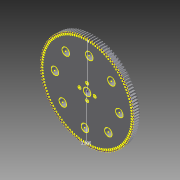
# Autodesk Inventor part: 120 tooth gear
Saved by Autodesk Inventor 2015 (Build 190159000, 159)
## iProperties
Created: 2011-10-31
Part Number: 120 tooth gear
Material: Generic
Document SubType Name: Modeling
Designer: Kyle
Density: 1 g/cm^3
Appearance: Default
Author: Kyle
Autodesk Inventor part; units mm, degrees
ref_plane "YZ Plane" through (0, 0, 0) normal (1, 0, 0) x (0, 1, 0)
ref_plane "XZ Plane" through (0, 0, 0) normal (0, 1, 0) x (-1, 0, 0)
ref_plane "XY Plane" through (0, 0, 0) normal (0, 0, 1) x (1, 0, 0)
sketch "Sketch1" plane through (0, 0, 0) normal (0, 0, 1) x (1, 0, 0)
  circle A0 centre (0, 0) radius 46.0375
  circle A1 centre (0, 0) radius 3.9688
  circle A2 centre (0, 7.9375) radius 1.5875
  circle A3 centre (-7.9375, 0) radius 1.5875
  circle A4 centre (0, -7.9375) radius 1.5875
  circle A5 centre (7.9375, 0) radius 1.5875
  circle A6 centre (25.4, 22.225) radius 3.9688
  circle A7 centre (0, 0) radius 3.9688
  circle A8 centre (2.2451, 33.676) radius 3.9688
  circle A9 centre (0, 0) radius 3.9688
  circle A10 centre (-22.225, 25.4) radius 3.9688
  circle A11 centre (0, 0) radius 3.9688
  circle A12 centre (-33.676, 2.2451) radius 3.9688
  circle A13 centre (0, 0) radius 3.9688
  circle A14 centre (-25.4, -22.225) radius 3.9688
  circle A15 centre (0, 0) radius 3.9688
  circle A16 centre (-2.2451, -33.676) radius 3.9688
  circle A17 centre (0, 0) radius 3.9688
  circle A18 centre (22.225, -25.4) radius 3.9688
  circle A19 centre (0, 0) radius 3.9688
  circle A20 centre (33.676, -2.2451) radius 3.9688
  dimension "d0" = 92.075
  dimension "d1" = 7.9375
  dimension "d2" = 3.175
  dimension "d3" = 7.9375
  dimension "d6" = 360
  dimension "d8" = 7.9375
  dimension "d9" = 22.225
  dimension "d10" = 25.4
  dimension "d13" = 360
  constraints: 21 centre point, 4 coincident, 40 other
  measures "d0" diameter of A0
  measures "d1" diameter of A1
  measures "d2" diameter of A2
  measures "d3" distance of A1.centre A2.centre
  measures "d8" diameter of A6
  measures "d9" vertical distance of A1.centre A6.centre
  measures "d10" horizontal distance of A1.centre A6.centre
extrude "Extrusion1" add sketch "Sketch1" along normal blind 6.35
sketch "Sketch2" plane through (0, 0, 6.35) normal (0, 0, 1) x (1, 0, 0)
  circle A0 centre (0, 0) radius 46.0375 projected
  line L0 (0, 46.0375) -> (0, 48.6765) construction
  line L1 (0, 48.6765) -> (0.3969, 48.6765)
  line L2 (0.3969, 48.6765) -> (0.7937, 47.089)
  line L3 (0.7937, 47.089) -> (0.7938, 46.0307)
  line L4 (0, 48.6765) -> (-0.3969, 48.6765)
  line L5 (-0.3969, 48.6765) -> (-0.7938, 47.089)
  line L6 (-0.7938, 47.089) -> (-0.7938, 46.0307)
  arc A1 (0.7938, 46.0307) -> (-0.7938, 46.0307) centre (0, 0) ccw
  dimension "d17" = 0.3969
  dimension "d18" = 1.5875
  dimension "d19" = 0.3969
  dimension "d20" = 1.0583
  constraints: 14 end point, 4 point on circle, 3 symmetric about line, 2 perpendicular, 1 centre point, 1 coincident, 1 concentric, 1 vertical
  measures "d17" distance of L0.end L1.end
  measures "d18" vertical distance of L1.end L2.end
  measures "d19" horizontal distance of L1.end L2.end
  measures "d20" distance of L2.end L3.end
extrude "Extrusion2" add sketch "Sketch2" against normal blind 6.35 contours A0 L6 L5 L4 L1 L2 L3
pattern_circular "Circular Pattern1" count 120 over 360 about axis through (0, 0, 0) along (0, 0, 1) of "Extrusion2"
sketch "Sketch3" plane through (0, 0, 6.35) normal (0, 0, 1) x (1, 0, 0)
  circle A0 centre (33.676, -2.2451) radius 3.9687 projected
  circle A1 centre (22.225, -25.4) radius 3.9687 projected
  circle A2 centre (-2.2451, -33.676) radius 3.9687 projected
  circle A3 centre (-25.4, -22.225) radius 3.9687 projected
  circle A4 centre (-33.676, 2.2451) radius 3.9687 projected
  circle A5 centre (-22.225, 25.4) radius 3.9687 projected
  circle A6 centre (2.2451, 33.676) radius 3.9687 projected
  circle A7 centre (25.4, 22.225) radius 3.9687 projected
  circle A8 centre (0, 0) radius 3.9687 projected
  circle A9 centre (7.9375, 0) radius 1.5875 projected
  circle A10 centre (0, -7.9375) radius 1.5875 projected
  circle A11 centre (-7.9375, 0) radius 1.5875 projected
  circle A12 centre (0, 7.9375) radius 1.5875 projected
  arc A13 (1.6164, 46.0091) -> (0.7938, 46.0307) centre (0, 0) ccw projected
  line L0 (0.7937, 47.089) -> (0.7938, 46.0307) projected
  line L1 (0.3969, 48.6765) -> (0.7937, 47.089) projected
  line L2 (-0.3969, 48.6765) -> (0.3969, 48.6765) projected
  line L3 (-0.7938, 47.089) -> (-0.3969, 48.6765) projected
  line L4 (-0.7938, 46.0307) -> (-0.7938, 47.089) projected
  arc A14 (-0.7938, 46.0307) -> (-1.6164, 46.0091) centre (0, 0) ccw projected
  line L5 (-1.6718, 47.066) -> (-1.6164, 46.0091) projected
  line L6 (-2.1512, 48.6306) -> (-1.6718, 47.066) projected
  line L7 (-2.9439, 48.589) -> (-2.1512, 48.6306) projected
  line L8 (-3.2571, 46.9829) -> (-2.9439, 48.589) projected
  line L9 (-3.2017, 45.926) -> (-3.2571, 46.9829) projected
  arc A15 (-3.2017, 45.926) -> (-4.0221, 45.8615) centre (0, 0) ccw projected
  line L10 (-4.1327, 46.914) -> (-4.0221, 45.8615) projected
  line L11 (-4.6934, 48.4513) -> (-4.1327, 46.914) projected
  line L12 (-5.4828, 48.3684) -> (-4.6934, 48.4513) projected
  line L13 (-5.7115, 46.7481) -> (-5.4828, 48.3684) projected
  line L14 (-5.6009, 45.6955) -> (-5.7115, 46.7481) projected
  arc A16 (-5.6009, 45.6955) -> (-6.4168, 45.5881) centre (0, 0) ccw projected
  line L15 (-6.5824, 46.6334) -> (-6.4168, 45.5881) projected
  line L16 (-7.2227, 48.1393) -> (-6.5824, 46.6334) projected
  line L17 (-8.0067, 48.0151) -> (-7.2227, 48.1393) projected
  line L18 (-8.1503, 46.3851) -> (-8.0067, 48.0151) projected
  line L19 (-7.9848, 45.3398) -> (-8.1503, 46.3851) projected
  arc A17 (-7.9848, 45.3398) -> (-8.7939, 45.1898) centre (0, 0) ccw projected
  line L20 (-9.0139, 46.225) -> (-8.7939, 45.1898) projected
  line L21 (-9.7322, 47.6953) -> (-9.0139, 46.225) projected
  line L22 (-10.5086, 47.5303) -> (-9.7322, 47.6953) projected
  line L23 (-10.5668, 45.895) -> (-10.5086, 47.5303) projected
  line L24 (-10.3467, 44.8597) -> (-10.5668, 45.895) projected
  arc A18 (-10.3467, 44.8597) -> (-11.1469, 44.6676) centre (0, 0) ccw projected
  line L25 (-11.4208, 45.6899) -> (-11.1469, 44.6676) projected
  line L26 (-12.2151, 47.1206) -> (-11.4208, 45.6899) projected
  line L27 (-12.9818, 46.9152) -> (-12.2151, 47.1206) projected
  line L28 (-12.9542, 45.279) -> (-12.9818, 46.9152) projected
  line L29 (-12.6803, 44.2568) -> (-12.9542, 45.279) projected
  arc A19 (-12.6803, 44.2568) -> (-13.4694, 44.023) centre (0, 0) ccw projected
  line L30 (-13.7964, 45.0296) -> (-13.4694, 44.023) projected
  line L31 (-14.6644, 46.4167) -> (-13.7964, 45.0296) projected
  line L32 (-15.4193, 46.1715) -> (-14.6644, 46.4167) projected
  line L33 (-15.3062, 44.539) -> (-15.4193, 46.1715) projected
  line L34 (-14.9792, 43.5325) -> (-15.3062, 44.539) projected
  arc A20 (-14.9792, 43.5325) -> (-15.7549, 43.2578) centre (0, 0) ccw projected
  line L35 (-16.1342, 44.2458) -> (-15.7549, 43.2578) projected
  line L36 (-17.0736, 45.5856) -> (-16.1342, 44.2458) projected
  line L37 (-17.8146, 45.3012) -> (-17.0736, 45.5856) projected
  line L38 (-17.6162, 43.6769) -> (-17.8146, 45.3012) projected
  line L39 (-17.2369, 42.6889) -> (-17.6162, 43.6769) projected
  arc A21 (-17.2369, 42.6889) -> (-17.9972, 42.3739) centre (0, 0) ccw projected
  line L40 (-18.4277, 43.3408) -> (-17.9972, 42.3739) projected
  line L41 (-19.4359, 44.6296) -> (-18.4277, 43.3408) projected
  line L42 (-20.1611, 44.3068) -> (-19.4359, 44.6296) projected
  line L43 (-19.8779, 42.6951) -> (-20.1611, 44.3068) projected
  line L44 (-19.4475, 41.7283) -> (-19.8779, 42.6951) projected
  arc A22 (-19.4475, 41.7283) -> (-20.1902, 41.374) centre (0, 0) ccw projected
  line L45 (-20.6707, 42.317) -> (-20.1902, 41.374) projected
  line L46 (-21.745, 43.5512) -> (-20.6707, 42.317) projected
  line L47 (-22.4523, 43.1909) -> (-21.745, 43.5512) projected
  line L48 (-22.0852, 41.5962) -> (-22.4523, 43.1909) projected
  line L49 (-21.6047, 40.6533) -> (-22.0852, 41.5962) projected
  arc A23 (-21.6047, 40.6533) -> (-22.3279, 40.2606) centre (0, 0) ccw projected
  line L50 (-22.8571, 41.1771) -> (-22.3279, 40.2606) projected
  line L51 (-23.9945, 42.3535) -> (-22.8571, 41.1771) projected
  line L52 (-24.6819, 41.9566) -> (-23.9945, 42.3535) projected
  line L53 (-24.2319, 40.3834) -> (-24.6819, 41.9566) projected
  line L54 (-23.7027, 39.4668) -> (-24.2319, 40.3834) projected
  arc A24 (-23.7027, 39.4668) -> (-24.4044, 39.0369) centre (0, 0) ccw projected
  line L55 (-24.9808, 39.9245) -> (-24.4044, 39.0369) projected
  line L56 (-26.1783, 41.0397) -> (-24.9808, 39.9245) projected
  line L57 (-26.844, 40.6074) -> (-26.1783, 41.0397) projected
  line L58 (-26.3122, 39.0598) -> (-26.844, 40.6074) projected
  line L59 (-25.7358, 38.1722) -> (-26.3122, 39.0598) projected
  arc A25 (-25.7358, 38.1722) -> (-26.414, 37.7061) centre (0, 0) ccw projected
  line L60 (-27.0361, 38.5623) -> (-26.414, 37.7061) projected
  line L61 (-28.2902, 39.6134) -> (-27.0361, 38.5623) projected
  line L62 (-28.9324, 39.1468) -> (-28.2902, 39.6134) projected
  line L63 (-28.3204, 37.6292) -> (-28.9324, 39.1468) projected
  line L64 (-27.6983, 36.773) -> (-28.3204, 37.6292) projected
  arc A26 (-27.6983, 36.773) -> (-28.3512, 36.2721) centre (0, 0) ccw projected
  line L65 (-29.0172, 37.0945) -> (-28.3512, 36.2721) projected
  line L66 (-30.3247, 38.0785) -> (-29.0172, 37.0945) projected
  line L67 (-30.9415, 37.579) -> (-30.3247, 38.0785) projected
  line L68 (-30.2509, 36.0955) -> (-30.9415, 37.579) projected
  line L69 (-29.5849, 35.273) -> (-30.2509, 36.0955) projected
  arc A27 (-29.5849, 35.273) -> (-30.2107, 34.7386) centre (0, 0) ccw projected
  line L70 (-30.9188, 35.5251) -> (-30.2107, 34.7386) projected
  line L71 (-32.276, 36.4392) -> (-30.9188, 35.5251) projected
  line L72 (-32.8659, 35.9081) -> (-32.276, 36.4392) projected
  line L73 (-32.0986, 34.4628) -> (-32.8659, 35.9081) projected
  line L74 (-31.3904, 33.6763) -> (-32.0986, 34.4628) projected
  arc A28 (-31.3904, 33.6763) -> (-31.9873, 33.1099) centre (0, 0) ccw projected
  line L75 (-32.7357, 33.8582) -> (-31.9873, 33.1099) projected
  line L76 (-34.1388, 34.7001) -> (-32.7357, 33.8582) projected
  line L77 (-34.7001, 34.1388) -> (-34.1388, 34.7001) projected
  line L78 (-33.8582, 32.7357) -> (-34.7001, 34.1388) projected
  line L79 (-33.1099, 31.9873) -> (-33.8582, 32.7357) projected
  arc A29 (-33.1099, 31.9873) -> (-33.6763, 31.3904) centre (0, 0) ccw projected
  line L80 (-34.4628, 32.0986) -> (-33.6763, 31.3904) projected
  line L81 (-35.9081, 32.8659) -> (-34.4628, 32.0986) projected
  line L82 (-36.4392, 32.276) -> (-35.9081, 32.8659) projected
  line L83 (-35.5251, 30.9188) -> (-36.4392, 32.276) projected
  line L84 (-34.7386, 30.2107) -> (-35.5251, 30.9188) projected
  arc A30 (-34.7386, 30.2107) -> (-35.273, 29.5849) centre (0, 0) ccw projected
  line L85 (-36.0955, 30.2509) -> (-35.273, 29.5849) projected
  line L86 (-37.579, 30.9415) -> (-36.0955, 30.2509) projected
  line L87 (-38.0785, 30.3247) -> (-37.579, 30.9415) projected
  line L88 (-37.0945, 29.0172) -> (-38.0785, 30.3247) projected
  line L89 (-36.2721, 28.3512) -> (-37.0945, 29.0172) projected
  arc A31 (-36.2721, 28.3512) -> (-36.773, 27.6983) centre (0, 0) ccw projected
  line L90 (-37.6292, 28.3204) -> (-36.773, 27.6983) projected
  line L91 (-39.1468, 28.9324) -> (-37.6292, 28.3204) projected
  line L92 (-39.6134, 28.2902) -> (-39.1468, 28.9324) projected
  line L93 (-38.5623, 27.0361) -> (-39.6134, 28.2902) projected
  line L94 (-37.7061, 26.414) -> (-38.5623, 27.0361) projected
  arc A32 (-37.7061, 26.414) -> (-38.1722, 25.7358) centre (0, 0) ccw projected
  line L95 (-39.0598, 26.3122) -> (-38.1722, 25.7358) projected
  line L96 (-40.6074, 26.844) -> (-39.0598, 26.3122) projected
  line L97 (-41.0397, 26.1783) -> (-40.6074, 26.844) projected
  line L98 (-39.9245, 24.9808) -> (-41.0397, 26.1783) projected
  line L99 (-39.0369, 24.4044) -> (-39.9245, 24.9808) projected
  arc A33 (-39.0369, 24.4044) -> (-39.4668, 23.7027) centre (0, 0) ccw projected
  line L100 (-40.3834, 24.2319) -> (-39.4668, 23.7027) projected
  line L101 (-41.9566, 24.6819) -> (-40.3834, 24.2319) projected
  line L102 (-42.3535, 23.9945) -> (-41.9566, 24.6819) projected
  line L103 (-41.1771, 22.8571) -> (-42.3535, 23.9945) projected
  line L104 (-40.2606, 22.3279) -> (-41.1771, 22.8571) projected
  arc A34 (-40.2606, 22.3279) -> (-40.6533, 21.6047) centre (0, 0) ccw projected
  line L105 (-41.5962, 22.0852) -> (-40.6533, 21.6047) projected
  line L106 (-43.1909, 22.4523) -> (-41.5962, 22.0852) projected
  line L107 (-43.5512, 21.745) -> (-43.1909, 22.4523) projected
  line L108 (-42.317, 20.6707) -> (-43.5512, 21.745) projected
  line L109 (-41.374, 20.1902) -> (-42.317, 20.6707) projected
  arc A35 (-41.374, 20.1902) -> (-41.7283, 19.4475) centre (0, 0) ccw projected
  line L110 (-42.6951, 19.8779) -> (-41.7283, 19.4475) projected
  line L111 (-44.3068, 20.1611) -> (-42.6951, 19.8779) projected
  line L112 (-44.6296, 19.4359) -> (-44.3068, 20.1611) projected
  line L113 (-43.3408, 18.4277) -> (-44.6296, 19.4359) projected
  line L114 (-42.3739, 17.9972) -> (-43.3408, 18.4277) projected
  arc A36 (-42.3739, 17.9972) -> (-42.6889, 17.2369) centre (0, 0) ccw projected
  line L115 (-43.6769, 17.6162) -> (-42.6889, 17.2369) projected
  line L116 (-45.3012, 17.8146) -> (-43.6769, 17.6162) projected
  line L117 (-45.5856, 17.0736) -> (-45.3012, 17.8146) projected
  line L118 (-44.2458, 16.1342) -> (-45.5856, 17.0736) projected
  line L119 (-43.2578, 15.7549) -> (-44.2458, 16.1342) projected
  arc A37 (-43.2578, 15.7549) -> (-43.5325, 14.9792) centre (0, 0) ccw projected
  line L120 (-44.539, 15.3062) -> (-43.5325, 14.9792) projected
  line L121 (-46.1715, 15.4193) -> (-44.539, 15.3062) projected
  line L122 (-46.4167, 14.6644) -> (-46.1715, 15.4193) projected
  line L123 (-45.0296, 13.7964) -> (-46.4167, 14.6644) projected
  line L124 (-44.023, 13.4694) -> (-45.0296, 13.7964) projected
  arc A38 (-44.023, 13.4694) -> (-44.2568, 12.6803) centre (0, 0) ccw projected
  line L125 (-45.279, 12.9542) -> (-44.2568, 12.6803) projected
  line L126 (-46.9152, 12.9818) -> (-45.279, 12.9542) projected
  line L127 (-47.1206, 12.2151) -> (-46.9152, 12.9818) projected
  line L128 (-45.6899, 11.4208) -> (-47.1206, 12.2151) projected
  line L129 (-44.6676, 11.1469) -> (-45.6899, 11.4208) projected
  arc A39 (-44.6676, 11.1469) -> (-44.8597, 10.3467) centre (0, 0) ccw projected
  line L130 (-45.895, 10.5668) -> (-44.8597, 10.3467) projected
  line L131 (-47.5303, 10.5086) -> (-45.895, 10.5668) projected
  line L132 (-47.6953, 9.7322) -> (-47.5303, 10.5086) projected
  line L133 (-46.225, 9.0139) -> (-47.6953, 9.7322) projected
  line L134 (-45.1898, 8.7939) -> (-46.225, 9.0139) projected
  arc A40 (-45.1898, 8.7939) -> (-45.3398, 7.9848) centre (0, 0) ccw projected
  line L135 (-46.3851, 8.1503) -> (-45.3398, 7.9848) projected
  line L136 (-48.0151, 8.0067) -> (-46.3851, 8.1503) projected
  line L137 (-48.1393, 7.2227) -> (-48.0151, 8.0067) projected
  line L138 (-46.6334, 6.5824) -> (-48.1393, 7.2227) projected
  line L139 (-45.5881, 6.4168) -> (-46.6334, 6.5824) projected
  arc A41 (-45.5881, 6.4168) -> (-45.6955, 5.6009) centre (0, 0) ccw projected
  line L140 (-46.7481, 5.7115) -> (-45.6955, 5.6009) projected
  line L141 (-48.3684, 5.4828) -> (-46.7481, 5.7115) projected
  line L142 (-48.4513, 4.6934) -> (-48.3684, 5.4828) projected
  line L143 (-46.914, 4.1327) -> (-48.4513, 4.6934) projected
  line L144 (-45.8615, 4.0221) -> (-46.914, 4.1327) projected
  arc A42 (-45.8615, 4.0221) -> (-45.926, 3.2017) centre (0, 0) ccw projected
  line L145 (-46.9829, 3.2571) -> (-45.926, 3.2017) projected
  line L146 (-48.589, 2.9439) -> (-46.9829, 3.2571) projected
  line L147 (-48.6306, 2.1512) -> (-48.589, 2.9439) projected
  line L148 (-47.066, 1.6718) -> (-48.6306, 2.1512) projected
  line L149 (-46.0091, 1.6164) -> (-47.066, 1.6718) projected
  arc A43 (-46.0091, 1.6164) -> (-46.0307, 0.7938) centre (0, 0) ccw projected
  line L150 (-47.089, 0.7938) -> (-46.0307, 0.7938) projected
  line L151 (-48.6765, 0.3969) -> (-47.089, 0.7938) projected
  line L152 (-48.6765, -0.3969) -> (-48.6765, 0.3969) projected
  line L153 (-47.089, -0.7937) -> (-48.6765, -0.3969) projected
  line L154 (-46.0307, -0.7937) -> (-47.089, -0.7937) projected
  arc A44 (-46.0307, -0.7937) -> (-46.0091, -1.6164) centre (0, 0) ccw projected
  line L155 (-47.066, -1.6718) -> (-46.0091, -1.6164) projected
  line L156 (-48.6306, -2.1512) -> (-47.066, -1.6718) projected
  line L157 (-48.589, -2.9439) -> (-48.6306, -2.1512) projected
  line L158 (-46.9829, -3.2571) -> (-48.589, -2.9439) projected
  line L159 (-45.926, -3.2017) -> (-46.9829, -3.2571) projected
  arc A45 (-45.926, -3.2017) -> (-45.8615, -4.0221) centre (0, 0) ccw projected
  line L160 (-46.914, -4.1327) -> (-45.8615, -4.0221) projected
  line L161 (-48.4513, -4.6934) -> (-46.914, -4.1327) projected
  line L162 (-48.3684, -5.4828) -> (-48.4513, -4.6934) projected
  line L163 (-46.7481, -5.7115) -> (-48.3684, -5.4828) projected
  line L164 (-45.6955, -5.6009) -> (-46.7481, -5.7115) projected
  arc A46 (-45.6955, -5.6009) -> (-45.5881, -6.4168) centre (0, 0) ccw projected
  line L165 (-46.6334, -6.5824) -> (-45.5881, -6.4168) projected
  line L166 (-48.1393, -7.2227) -> (-46.6334, -6.5824) projected
  line L167 (-48.0151, -8.0067) -> (-48.1393, -7.2227) projected
  line L168 (-46.3851, -8.1503) -> (-48.0151, -8.0067) projected
  line L169 (-45.3398, -7.9848) -> (-46.3851, -8.1503) projected
  arc A47 (-45.3398, -7.9848) -> (-45.1898, -8.7939) centre (0, 0) ccw projected
  line L170 (-46.225, -9.0139) -> (-45.1898, -8.7939) projected
  line L171 (-47.6953, -9.7322) -> (-46.225, -9.0139) projected
  line L172 (-47.5303, -10.5086) -> (-47.6953, -9.7322) projected
  line L173 (-45.895, -10.5668) -> (-47.5303, -10.5086) projected
  line L174 (-44.8597, -10.3467) -> (-45.895, -10.5668) projected
  arc A48 (-44.8597, -10.3467) -> (-44.6676, -11.1469) centre (0, 0) ccw projected
  line L175 (-45.6899, -11.4208) -> (-44.6676, -11.1469) projected
  line L176 (-47.1206, -12.2151) -> (-45.6899, -11.4208) projected
  line L177 (-46.9152, -12.9818) -> (-47.1206, -12.2151) projected
  line L178 (-45.279, -12.9542) -> (-46.9152, -12.9818) projected
  line L179 (-44.2568, -12.6803) -> (-45.279, -12.9542) projected
  arc A49 (-44.2568, -12.6803) -> (-44.023, -13.4694) centre (0, 0) ccw projected
  line L180 (-45.0296, -13.7964) -> (-44.023, -13.4694) projected
  line L181 (-46.4167, -14.6644) -> (-45.0296, -13.7964) projected
  line L182 (-46.1715, -15.4193) -> (-46.4167, -14.6644) projected
  line L183 (-44.539, -15.3062) -> (-46.1715, -15.4193) projected
  line L184 (-43.5325, -14.9792) -> (-44.539, -15.3062) projected
  arc A50 (-43.5325, -14.9792) -> (-43.2578, -15.7549) centre (0, 0) ccw projected
  line L185 (-44.2458, -16.1342) -> (-43.2578, -15.7549) projected
  line L186 (-45.5856, -17.0736) -> (-44.2458, -16.1342) projected
  line L187 (-45.3012, -17.8146) -> (-45.5856, -17.0736) projected
  line L188 (-43.6769, -17.6162) -> (-45.3012, -17.8146) projected
  line L189 (-42.6889, -17.2369) -> (-43.6769, -17.6162) projected
  arc A51 (-42.6889, -17.2369) -> (-42.3739, -17.9972) centre (0, 0) ccw projected
  line L190 (-43.3408, -18.4277) -> (-42.3739, -17.9972) projected
  line L191 (-44.6296, -19.4359) -> (-43.3408, -18.4277) projected
  line L192 (-44.3068, -20.1611) -> (-44.6296, -19.4359) projected
  line L193 (-42.6951, -19.8779) -> (-44.3068, -20.1611) projected
  line L194 (-41.7283, -19.4475) -> (-42.6951, -19.8779) projected
  arc A52 (-41.7283, -19.4475) -> (-41.374, -20.1902) centre (0, 0) ccw projected
  line L195 (-42.317, -20.6707) -> (-41.374, -20.1902) projected
  line L196 (-43.5512, -21.745) -> (-42.317, -20.6707) projected
  line L197 (-43.1909, -22.4523) -> (-43.5512, -21.745) projected
  line L198 (-41.5962, -22.0852) -> (-43.1909, -22.4523) projected
  line L199 (-40.6533, -21.6047) -> (-41.5962, -22.0852) projected
  arc A53 (-40.6533, -21.6047) -> (-40.2606, -22.3279) centre (0, 0) ccw projected
  line L200 (-41.1771, -22.8571) -> (-40.2606, -22.3279) projected
  line L201 (-42.3535, -23.9945) -> (-41.1771, -22.8571) projected
  line L202 (-41.9566, -24.6819) -> (-42.3535, -23.9945) projected
  line L203 (-40.3834, -24.2319) -> (-41.9566, -24.6819) projected
  line L204 (-39.4668, -23.7027) -> (-40.3834, -24.2319) projected
  arc A54 (-39.4668, -23.7027) -> (-39.0369, -24.4044) centre (0, 0) ccw projected
  line L205 (-39.9245, -24.9808) -> (-39.0369, -24.4044) projected
  line L206 (-41.0397, -26.1783) -> (-39.9245, -24.9808) projected
  line L207 (-40.6074, -26.844) -> (-41.0397, -26.1783) projected
  line L208 (-39.0598, -26.3122) -> (-40.6074, -26.844) projected
  line L209 (-38.1722, -25.7358) -> (-39.0598, -26.3122) projected
  arc A55 (-38.1722, -25.7358) -> (-37.7061, -26.414) centre (0, 0) ccw projected
  line L210 (-38.5623, -27.0361) -> (-37.7061, -26.414) projected
  line L211 (-39.6134, -28.2902) -> (-38.5623, -27.0361) projected
  line L212 (-39.1468, -28.9324) -> (-39.6134, -28.2902) projected
  line L213 (-37.6292, -28.3204) -> (-39.1468, -28.9324) projected
  line L214 (-36.773, -27.6983) -> (-37.6292, -28.3204) projected
  arc A56 (-36.773, -27.6983) -> (-36.2721, -28.3512) centre (0, 0) ccw projected
  line L215 (-37.0945, -29.0172) -> (-36.2721, -28.3512) projected
  line L216 (-38.0785, -30.3247) -> (-37.0945, -29.0172) projected
  line L217 (-37.579, -30.9415) -> (-38.0785, -30.3247) projected
  line L218 (-36.0955, -30.2509) -> (-37.579, -30.9415) projected
  line L219 (-35.273, -29.5849) -> (-36.0955, -30.2509) projected
  arc A57 (-35.273, -29.5849) -> (-34.7386, -30.2107) centre (0, 0) ccw projected
  line L220 (-35.5251, -30.9188) -> (-34.7386, -30.2107) projected
  line L221 (-36.4392, -32.276) -> (-35.5251, -30.9188) projected
  line L222 (-35.9081, -32.8659) -> (-36.4392, -32.276) projected
  line L223 (-34.4628, -32.0986) -> (-35.9081, -32.8659) projected
  line L224 (-33.6763, -31.3904) -> (-34.4628, -32.0986) projected
  arc A58 (-33.6763, -31.3904) -> (-33.1099, -31.9873) centre (0, 0) ccw projected
  line L225 (-33.8582, -32.7357) -> (-33.1099, -31.9873) projected
  line L226 (-34.7001, -34.1388) -> (-33.8582, -32.7357) projected
  line L227 (-34.1388, -34.7001) -> (-34.7001, -34.1388) projected
  line L228 (-32.7357, -33.8582) -> (-34.1388, -34.7001) projected
  line L229 (-31.9873, -33.1099) -> (-32.7357, -33.8582) projected
  arc A59 (-31.9873, -33.1099) -> (-31.3904, -33.6763) centre (0, 0) ccw projected
  line L230 (-32.0986, -34.4628) -> (-31.3904, -33.6763) projected
  line L231 (-32.8659, -35.9081) -> (-32.0986, -34.4628) projected
  line L232 (-32.276, -36.4392) -> (-32.8659, -35.9081) projected
  line L233 (-30.9188, -35.5251) -> (-32.276, -36.4392) projected
  line L234 (-30.2107, -34.7386) -> (-30.9188, -35.5251) projected
  arc A60 (-30.2107, -34.7386) -> (-29.5849, -35.273) centre (0, 0) ccw projected
  line L235 (-30.2509, -36.0955) -> (-29.5849, -35.273) projected
  line L236 (-30.9415, -37.579) -> (-30.2509, -36.0955) projected
  line L237 (-30.3247, -38.0785) -> (-30.9415, -37.579) projected
  line L238 (-29.0172, -37.0945) -> (-30.3247, -38.0785) projected
  line L239 (-28.3512, -36.2721) -> (-29.0172, -37.0945) projected
  arc A61 (-28.3512, -36.2721) -> (-27.6983, -36.773) centre (0, 0) ccw projected
  line L240 (-28.3204, -37.6292) -> (-27.6983, -36.773) projected
  line L241 (-28.9324, -39.1468) -> (-28.3204, -37.6292) projected
  line L242 (-28.2902, -39.6134) -> (-28.9324, -39.1468) projected
  line L243 (-27.0361, -38.5623) -> (-28.2902, -39.6134) projected
  line L244 (-26.414, -37.7061) -> (-27.0361, -38.5623) projected
  arc A62 (-26.414, -37.7061) -> (-25.7358, -38.1722) centre (0, 0) ccw projected
  line L245 (-26.3122, -39.0598) -> (-25.7358, -38.1722) projected
  line L246 (-26.844, -40.6074) -> (-26.3122, -39.0598) projected
  line L247 (-26.1783, -41.0397) -> (-26.844, -40.6074) projected
  line L248 (-24.9808, -39.9245) -> (-26.1783, -41.0397) projected
  line L249 (-24.4044, -39.0369) -> (-24.9808, -39.9245) projected
  arc A63 (-24.4044, -39.0369) -> (-23.7027, -39.4668) centre (0, 0) ccw projected
  line L250 (-24.2319, -40.3834) -> (-23.7027, -39.4668) projected
  line L251 (-24.6819, -41.9566) -> (-24.2319, -40.3834) projected
  line L252 (-23.9945, -42.3535) -> (-24.6819, -41.9566) projected
  line L253 (-22.8571, -41.1771) -> (-23.9945, -42.3535) projected
  line L254 (-22.3279, -40.2606) -> (-22.8571, -41.1771) projected
  arc A64 (-22.3279, -40.2606) -> (-21.6047, -40.6533) centre (0, 0) ccw projected
  line L255 (-22.0852, -41.5962) -> (-21.6047, -40.6533) projected
  line L256 (-22.4523, -43.1909) -> (-22.0852, -41.5962) projected
  line L257 (-21.745, -43.5512) -> (-22.4523, -43.1909) projected
  line L258 (-20.6707, -42.317) -> (-21.745, -43.5512) projected
  line L259 (-20.1902, -41.374) -> (-20.6707, -42.317) projected
  arc A65 (-20.1902, -41.374) -> (-19.4475, -41.7283) centre (0, 0) ccw projected
  line L260 (-19.8779, -42.6951) -> (-19.4475, -41.7283) projected
  line L261 (-20.1611, -44.3068) -> (-19.8779, -42.6951) projected
  line L262 (-19.4359, -44.6296) -> (-20.1611, -44.3068) projected
  line L263 (-18.4277, -43.3408) -> (-19.4359, -44.6296) projected
  line L264 (-17.9972, -42.3739) -> (-18.4277, -43.3408) projected
  arc A66 (-17.9972, -42.3739) -> (-17.2369, -42.6889) centre (0, 0) ccw projected
  line L265 (-17.6162, -43.6769) -> (-17.2369, -42.6889) projected
  line L266 (-17.8146, -45.3012) -> (-17.6162, -43.6769) projected
  line L267 (-17.0736, -45.5856) -> (-17.8146, -45.3012) projected
  line L268 (-16.1342, -44.2458) -> (-17.0736, -45.5856) projected
  line L269 (-15.7549, -43.2578) -> (-16.1342, -44.2458) projected
  arc A67 (-15.7549, -43.2578) -> (-14.9792, -43.5325) centre (0, 0) ccw projected
  line L270 (-15.3062, -44.539) -> (-14.9792, -43.5325) projected
  line L271 (-15.4193, -46.1715) -> (-15.3062, -44.539) projected
  line L272 (-14.6644, -46.4167) -> (-15.4193, -46.1715) projected
  line L273 (-13.7964, -45.0296) -> (-14.6644, -46.4167) projected
  line L274 (-13.4694, -44.023) -> (-13.7964, -45.0296) projected
  arc A68 (-13.4694, -44.023) -> (-12.6803, -44.2568) centre (0, 0) ccw projected
  line L275 (-12.9542, -45.279) -> (-12.6803, -44.2568) projected
  line L276 (-12.9818, -46.9152) -> (-12.9542, -45.279) projected
  line L277 (-12.2151, -47.1206) -> (-12.9818, -46.9152) projected
  line L278 (-11.4208, -45.6899) -> (-12.2151, -47.1206) projected
  line L279 (-11.1469, -44.6676) -> (-11.4208, -45.6899) projected
  arc A69 (-11.1469, -44.6676) -> (-10.3467, -44.8597) centre (0, 0) ccw projected
  line L280 (-10.5668, -45.895) -> (-10.3467, -44.8597) projected
  line L281 (-10.5086, -47.5303) -> (-10.5668, -45.895) projected
  line L282 (-9.7322, -47.6953) -> (-10.5086, -47.5303) projected
  line L283 (-9.0139, -46.225) -> (-9.7322, -47.6953) projected
  line L284 (-8.7939, -45.1898) -> (-9.0139, -46.225) projected
  arc A70 (-8.7939, -45.1898) -> (-7.9848, -45.3398) centre (0, 0) ccw projected
  line L285 (-8.1503, -46.3851) -> (-7.9848, -45.3398) projected
  line L286 (-8.0067, -48.0151) -> (-8.1503, -46.3851) projected
  line L287 (-7.2227, -48.1393) -> (-8.0067, -48.0151) projected
  line L288 (-6.5824, -46.6334) -> (-7.2227, -48.1393) projected
  line L289 (-6.4168, -45.5881) -> (-6.5824, -46.6334) projected
  arc A71 (-6.4168, -45.5881) -> (-5.6009, -45.6955) centre (0, 0) ccw projected
  line L290 (-5.7115, -46.7481) -> (-5.6009, -45.6955) projected
  line L291 (-5.4828, -48.3684) -> (-5.7115, -46.7481) projected
  line L292 (-4.6934, -48.4513) -> (-5.4828, -48.3684) projected
  line L293 (-4.1327, -46.914) -> (-4.6934, -48.4513) projected
  line L294 (-4.0221, -45.8615) -> (-4.1327, -46.914) projected
  arc A72 (-4.0221, -45.8615) -> (-3.2017, -45.926) centre (0, 0) ccw projected
  line L295 (-3.2571, -46.9829) -> (-3.2017, -45.926) projected
  line L296 (-2.9439, -48.589) -> (-3.2571, -46.9829) projected
  line L297 (-2.1512, -48.6306) -> (-2.9439, -48.589) projected
  line L298 (-1.6718, -47.066) -> (-2.1512, -48.6306) projected
  line L299 (-1.6164, -46.0091) -> (-1.6718, -47.066) projected
  arc A73 (-1.6164, -46.0091) -> (-0.7938, -46.0307) centre (0, 0) ccw projected
  line L300 (-0.7938, -47.089) -> (-0.7938, -46.0307) projected
  line L301 (-0.3969, -48.6765) -> (-0.7938, -47.089) projected
  line L302 (0.3969, -48.6765) -> (-0.3969, -48.6765) projected
  line L303 (0.7937, -47.089) -> (0.3969, -48.6765) projected
  line L304 (0.7937, -46.0307) -> (0.7937, -47.089) projected
  arc A74 (0.7937, -46.0307) -> (1.6164, -46.0091) centre (0, 0) ccw projected
  line L305 (1.6718, -47.066) -> (1.6164, -46.0091) projected
  line L306 (2.1512, -48.6306) -> (1.6718, -47.066) projected
  line L307 (2.9439, -48.589) -> (2.1512, -48.6306) projected
  line L308 (3.2571, -46.9829) -> (2.9439, -48.589) projected
  line L309 (3.2017, -45.926) -> (3.2571, -46.9829) projected
  arc A75 (3.2017, -45.926) -> (4.0221, -45.8615) centre (0, 0) ccw projected
  line L310 (4.1327, -46.914) -> (4.0221, -45.8615) projected
  line L311 (4.6934, -48.4513) -> (4.1327, -46.914) projected
  line L312 (5.4828, -48.3684) -> (4.6934, -48.4513) projected
  line L313 (5.7115, -46.7481) -> (5.4828, -48.3684) projected
  line L314 (5.6009, -45.6955) -> (5.7115, -46.7481) projected
  arc A76 (5.6009, -45.6955) -> (6.4168, -45.5881) centre (0, 0) ccw projected
  line L315 (6.5824, -46.6334) -> (6.4168, -45.5881) projected
  line L316 (7.2227, -48.1393) -> (6.5824, -46.6334) projected
  line L317 (8.0067, -48.0151) -> (7.2227, -48.1393) projected
  line L318 (8.1503, -46.3851) -> (8.0067, -48.0151) projected
  line L319 (7.9848, -45.3398) -> (8.1503, -46.3851) projected
  arc A77 (7.9848, -45.3398) -> (8.7939, -45.1898) centre (0, 0) ccw projected
  line L320 (9.0139, -46.225) -> (8.7939, -45.1898) projected
  line L321 (9.7322, -47.6953) -> (9.0139, -46.225) projected
  line L322 (10.5086, -47.5303) -> (9.7322, -47.6953) projected
  line L323 (10.5668, -45.895) -> (10.5086, -47.5303) projected
  line L324 (10.3467, -44.8597) -> (10.5668, -45.895) projected
  arc A78 (10.3467, -44.8597) -> (11.1469, -44.6676) centre (0, 0) ccw projected
  line L325 (11.4208, -45.6899) -> (11.1469, -44.6676) projected
  line L326 (12.2151, -47.1206) -> (11.4208, -45.6899) projected
  line L327 (12.9818, -46.9152) -> (12.2151, -47.1206) projected
  line L328 (12.9542, -45.279) -> (12.9818, -46.9152) projected
  line L329 (12.6803, -44.2568) -> (12.9542, -45.279) projected
  arc A79 (12.6803, -44.2568) -> (13.4694, -44.023) centre (0, 0) ccw projected
  line L330 (13.7964, -45.0296) -> (13.4694, -44.023) projected
  line L331 (14.6644, -46.4167) -> (13.7964, -45.0296) projected
  line L332 (15.4193, -46.1715) -> (14.6644, -46.4167) projected
  line L333 (15.3062, -44.539) -> (15.4193, -46.1715) projected
  line L334 (14.9792, -43.5325) -> (15.3062, -44.539) projected
  arc A80 (14.9792, -43.5325) -> (15.7549, -43.2578) centre (0, 0) ccw projected
  line L335 (16.1342, -44.2458) -> (15.7549, -43.2578) projected
  line L336 (17.0736, -45.5856) -> (16.1342, -44.2458) projected
  line L337 (17.8146, -45.3012) -> (17.0736, -45.5856) projected
  line L338 (17.6162, -43.6769) -> (17.8146, -45.3012) projected
  line L339 (17.2369, -42.6889) -> (17.6162, -43.6769) projected
  arc A81 (17.2369, -42.6889) -> (17.9972, -42.3739) centre (0, 0) ccw projected
  line L340 (18.4277, -43.3408) -> (17.9972, -42.3739) projected
  line L341 (19.4359, -44.6296) -> (18.4277, -43.3408) projected
  line L342 (20.1611, -44.3068) -> (19.4359, -44.6296) projected
  line L343 (19.8779, -42.6951) -> (20.1611, -44.3068) projected
  line L344 (19.4475, -41.7283) -> (19.8779, -42.6951) projected
  arc A82 (19.4475, -41.7283) -> (20.1902, -41.374) centre (0, 0) ccw projected
  line L345 (20.6707, -42.317) -> (20.1902, -41.374) projected
  line L346 (21.745, -43.5512) -> (20.6707, -42.317) projected
  line L347 (22.4523, -43.1909) -> (21.745, -43.5512) projected
  line L348 (22.0852, -41.5962) -> (22.4523, -43.1909) projected
  line L349 (21.6047, -40.6533) -> (22.0852, -41.5962) projected
  arc A83 (21.6047, -40.6533) -> (22.3279, -40.2606) centre (0, 0) ccw projected
  line L350 (22.8571, -41.1771) -> (22.3279, -40.2606) projected
  line L351 (23.9945, -42.3535) -> (22.8571, -41.1771) projected
  line L352 (24.6819, -41.9566) -> (23.9945, -42.3535) projected
  line L353 (24.2319, -40.3834) -> (24.6819, -41.9566) projected
  line L354 (23.7027, -39.4668) -> (24.2319, -40.3834) projected
  arc A84 (23.7027, -39.4668) -> (24.4044, -39.0369) centre (0, 0) ccw projected
  line L355 (24.9808, -39.9245) -> (24.4044, -39.0369) projected
  line L356 (26.1783, -41.0397) -> (24.9808, -39.9245) projected
  line L357 (26.844, -40.6074) -> (26.1783, -41.0397) projected
  line L358 (26.3122, -39.0598) -> (26.844, -40.6074) projected
  line L359 (25.7358, -38.1722) -> (26.3122, -39.0598) projected
  arc A85 (25.7358, -38.1722) -> (26.414, -37.7061) centre (0, 0) ccw projected
  line L360 (27.0361, -38.5623) -> (26.414, -37.7061) projected
  line L361 (28.2902, -39.6134) -> (27.0361, -38.5623) projected
  line L362 (28.9324, -39.1468) -> (28.2902, -39.6134) projected
  line L363 (28.3204, -37.6292) -> (28.9324, -39.1468) projected
  line L364 (27.6983, -36.773) -> (28.3204, -37.6292) projected
  arc A86 (27.6983, -36.773) -> (28.3512, -36.2721) centre (0, 0) ccw projected
  line L365 (29.0172, -37.0945) -> (28.3512, -36.2721) projected
  line L366 (30.3247, -38.0785) -> (29.0172, -37.0945) projected
  line L367 (30.9415, -37.579) -> (30.3247, -38.0785) projected
  line L368 (30.2509, -36.0955) -> (30.9415, -37.579) projected
  line L369 (29.5849, -35.273) -> (30.2509, -36.0955) projected
  arc A87 (29.5849, -35.273) -> (30.2107, -34.7386) centre (0, 0) ccw projected
  line L370 (30.9188, -35.5251) -> (30.2107, -34.7386) projected
  line L371 (32.276, -36.4392) -> (30.9188, -35.5251) projected
  line L372 (32.8659, -35.9081) -> (32.276, -36.4392) projected
  line L373 (32.0986, -34.4628) -> (32.8659, -35.9081) projected
  line L374 (31.3904, -33.6763) -> (32.0986, -34.4628) projected
  arc A88 (31.3904, -33.6763) -> (31.9873, -33.1099) centre (0, 0) ccw projected
  line L375 (32.7357, -33.8582) -> (31.9873, -33.1099) projected
  line L376 (34.1388, -34.7001) -> (32.7357, -33.8582) projected
  line L377 (34.7001, -34.1388) -> (34.1388, -34.7001) projected
  line L378 (33.8582, -32.7357) -> (34.7001, -34.1388) projected
  line L379 (33.1099, -31.9873) -> (33.8582, -32.7357) projected
  arc A89 (33.1099, -31.9873) -> (33.6763, -31.3904) centre (0, 0) ccw projected
  line L380 (34.4628, -32.0986) -> (33.6763, -31.3904) projected
  line L381 (35.9081, -32.8659) -> (34.4628, -32.0986) projected
  line L382 (36.4392, -32.276) -> (35.9081, -32.8659) projected
  line L383 (35.5251, -30.9188) -> (36.4392, -32.276) projected
  line L384 (34.7386, -30.2107) -> (35.5251, -30.9188) projected
  arc A90 (34.7386, -30.2107) -> (35.273, -29.5849) centre (0, 0) ccw projected
  line L385 (36.0955, -30.2509) -> (35.273, -29.5849) projected
  line L386 (37.579, -30.9415) -> (36.0955, -30.2509) projected
  line L387 (38.0785, -30.3247) -> (37.579, -30.9415) projected
  line L388 (37.0945, -29.0172) -> (38.0785, -30.3247) projected
  line L389 (36.2721, -28.3512) -> (37.0945, -29.0172) projected
  arc A91 (36.2721, -28.3512) -> (36.773, -27.6983) centre (0, 0) ccw projected
  line L390 (37.6292, -28.3204) -> (36.773, -27.6983) projected
  line L391 (39.1468, -28.9324) -> (37.6292, -28.3204) projected
  line L392 (39.6134, -28.2902) -> (39.1468, -28.9324) projected
  line L393 (38.5623, -27.0361) -> (39.6134, -28.2902) projected
  line L394 (37.7061, -26.414) -> (38.5623, -27.0361) projected
  arc A92 (37.7061, -26.414) -> (38.1722, -25.7358) centre (0, 0) ccw projected
  line L395 (39.0598, -26.3122) -> (38.1722, -25.7358) projected
  line L396 (40.6074, -26.844) -> (39.0598, -26.3122) projected
  line L397 (41.0397, -26.1783) -> (40.6074, -26.844) projected
  line L398 (39.9245, -24.9808) -> (41.0397, -26.1783) projected
  line L399 (39.0369, -24.4044) -> (39.9245, -24.9808) projected
  arc A93 (39.0369, -24.4044) -> (39.4668, -23.7027) centre (0, 0) ccw projected
  line L400 (40.3834, -24.2319) -> (39.4668, -23.7027) projected
  line L401 (41.9566, -24.6819) -> (40.3834, -24.2319) projected
  line L402 (42.3535, -23.9945) -> (41.9566, -24.6819) projected
  line L403 (41.1771, -22.8571) -> (42.3535, -23.9945) projected
  line L404 (40.2606, -22.3279) -> (41.1771, -22.8571) projected
  arc A94 (40.2606, -22.3279) -> (40.6533, -21.6047) centre (0, 0) ccw projected
  line L405 (41.5962, -22.0852) -> (40.6533, -21.6047) projected
  line L406 (43.1909, -22.4523) -> (41.5962, -22.0852) projected
  line L407 (43.5512, -21.745) -> (43.1909, -22.4523) projected
  line L408 (42.317, -20.6707) -> (43.5512, -21.745) projected
  line L409 (41.374, -20.1902) -> (42.317, -20.6707) projected
  arc A95 (41.374, -20.1902) -> (41.7283, -19.4475) centre (0, 0) ccw projected
  line L410 (42.6951, -19.8779) -> (41.7283, -19.4475) projected
  line L411 (44.3068, -20.1611) -> (42.6951, -19.8779) projected
  line L412 (44.6296, -19.4359) -> (44.3068, -20.1611) projected
  line L413 (43.3408, -18.4277) -> (44.6296, -19.4359) projected
  line L414 (42.3739, -17.9972) -> (43.3408, -18.4277) projected
  arc A96 (42.3739, -17.9972) -> (42.6889, -17.2369) centre (0, 0) ccw projected
  line L415 (43.6769, -17.6162) -> (42.6889, -17.2369) projected
  line L416 (45.3012, -17.8146) -> (43.6769, -17.6162) projected
  line L417 (45.5856, -17.0736) -> (45.3012, -17.8146) projected
  line L418 (44.2458, -16.1342) -> (45.5856, -17.0736) projected
  line L419 (43.2578, -15.7549) -> (44.2458, -16.1342) projected
  arc A97 (43.2578, -15.7549) -> (43.5325, -14.9792) centre (0, 0) ccw projected
  line L420 (44.539, -15.3062) -> (43.5325, -14.9792) projected
  line L421 (46.1715, -15.4193) -> (44.539, -15.3062) projected
  line L422 (46.4167, -14.6644) -> (46.1715, -15.4193) projected
  line L423 (45.0296, -13.7964) -> (46.4167, -14.6644) projected
  line L424 (44.023, -13.4694) -> (45.0296, -13.7964) projected
  arc A98 (44.023, -13.4694) -> (44.2568, -12.6803) centre (0, 0) ccw projected
  line L425 (45.279, -12.9542) -> (44.2568, -12.6803) projected
  line L426 (46.9152, -12.9818) -> (45.279, -12.9542) projected
  line L427 (47.1206, -12.2151) -> (46.9152, -12.9818) projected
  line L428 (45.6899, -11.4208) -> (47.1206, -12.2151) projected
  line L429 (44.6676, -11.1469) -> (45.6899, -11.4208) projected
  arc A99 (44.6676, -11.1469) -> (44.8597, -10.3467) centre (0, 0) ccw projected
  line L430 (45.895, -10.5668) -> (44.8597, -10.3467) projected
  line L431 (47.5303, -10.5086) -> (45.895, -10.5668) projected
  line L432 (47.6953, -9.7322) -> (47.5303, -10.5086) projected
  line L433 (46.225, -9.0139) -> (47.6953, -9.7322) projected
  line L434 (45.1898, -8.7939) -> (46.225, -9.0139) projected
  arc A100 (45.1898, -8.7939) -> (45.3398, -7.9848) centre (0, 0) ccw projected
  line L435 (46.3851, -8.1503) -> (45.3398, -7.9848) projected
  line L436 (48.0151, -8.0067) -> (46.3851, -8.1503) projected
  line L437 (48.1393, -7.2227) -> (48.0151, -8.0067) projected
  line L438 (46.6334, -6.5824) -> (48.1393, -7.2227) projected
  line L439 (45.5881, -6.4168) -> (46.6334, -6.5824) projected
  arc A101 (45.5881, -6.4168) -> (45.6955, -5.6009) centre (0, 0) ccw projected
  line L440 (46.7481, -5.7115) -> (45.6955, -5.6009) projected
  line L441 (48.3684, -5.4828) -> (46.7481, -5.7115) projected
  line L442 (48.4513, -4.6934) -> (48.3684, -5.4828) projected
  line L443 (46.914, -4.1327) -> (48.4513, -4.6934) projected
  line L444 (45.8615, -4.0221) -> (46.914, -4.1327) projected
  arc A102 (45.8615, -4.0221) -> (45.926, -3.2017) centre (0, 0) ccw projected
  line L445 (46.9829, -3.2571) -> (45.926, -3.2017) projected
  line L446 (48.589, -2.9439) -> (46.9829, -3.2571) projected
  line L447 (48.6306, -2.1512) -> (48.589, -2.9439) projected
  line L448 (47.066, -1.6718) -> (48.6306, -2.1512) projected
  line L449 (46.0091, -1.6164) -> (47.066, -1.6718) projected
  arc A103 (46.0091, -1.6164) -> (46.0307, -0.7938) centre (0, 0) ccw projected
  line L450 (47.089, -0.7938) -> (46.0307, -0.7938) projected
  line L451 (48.6765, -0.3969) -> (47.089, -0.7938) projected
  line L452 (48.6765, 0.3969) -> (48.6765, -0.3969) projected
  line L453 (47.089, 0.7937) -> (48.6765, 0.3969) projected
  line L454 (46.0307, 0.7937) -> (47.089, 0.7937) projected
  arc A104 (46.0307, 0.7937) -> (46.0091, 1.6164) centre (0, 0) ccw projected
  line L455 (47.066, 1.6718) -> (46.0091, 1.6164) projected
  line L456 (48.6306, 2.1512) -> (47.066, 1.6718) projected
  line L457 (48.589, 2.9439) -> (48.6306, 2.1512) projected
  line L458 (46.9829, 3.2571) -> (48.589, 2.9439) projected
  line L459 (45.926, 3.2017) -> (46.9829, 3.2571) projected
  arc A105 (45.926, 3.2017) -> (45.8615, 4.0221) centre (0, 0) ccw projected
  line L460 (46.914, 4.1327) -> (45.8615, 4.0221) projected
  line L461 (48.4513, 4.6934) -> (46.914, 4.1327) projected
  line L462 (48.3684, 5.4828) -> (48.4513, 4.6934) projected
  line L463 (46.7481, 5.7115) -> (48.3684, 5.4828) projected
  line L464 (45.6955, 5.6009) -> (46.7481, 5.7115) projected
  arc A106 (45.6955, 5.6009) -> (45.5881, 6.4168) centre (0, 0) ccw projected
  line L465 (46.6334, 6.5824) -> (45.5881, 6.4168) projected
  line L466 (48.1393, 7.2227) -> (46.6334, 6.5824) projected
  line L467 (48.0151, 8.0067) -> (48.1393, 7.2227) projected
  line L468 (46.3851, 8.1503) -> (48.0151, 8.0067) projected
  line L469 (45.3398, 7.9848) -> (46.3851, 8.1503) projected
  arc A107 (45.3398, 7.9848) -> (45.1898, 8.7939) centre (0, 0) ccw projected
  line L470 (46.225, 9.0139) -> (45.1898, 8.7939) projected
  line L471 (47.6953, 9.7322) -> (46.225, 9.0139) projected
  line L472 (47.5303, 10.5086) -> (47.6953, 9.7322) projected
  line L473 (45.895, 10.5668) -> (47.5303, 10.5086) projected
  line L474 (44.8597, 10.3467) -> (45.895, 10.5668) projected
  arc A108 (44.8597, 10.3467) -> (44.6676, 11.1469) centre (0, 0) ccw projected
  line L475 (45.6899, 11.4208) -> (44.6676, 11.1469) projected
  line L476 (47.1206, 12.2151) -> (45.6899, 11.4208) projected
  line L477 (46.9152, 12.9818) -> (47.1206, 12.2151) projected
  line L478 (45.279, 12.9542) -> (46.9152, 12.9818) projected
  line L479 (44.2568, 12.6803) -> (45.279, 12.9542) projected
  arc A109 (44.2568, 12.6803) -> (44.023, 13.4694) centre (0, 0) ccw projected
  line L480 (45.0296, 13.7964) -> (44.023, 13.4694) projected
  line L481 (46.4167, 14.6644) -> (45.0296, 13.7964) projected
  line L482 (46.1715, 15.4193) -> (46.4167, 14.6644) projected
  line L483 (44.539, 15.3062) -> (46.1715, 15.4193) projected
  line L484 (43.5325, 14.9792) -> (44.539, 15.3062) projected
  arc A110 (43.5325, 14.9792) -> (43.2578, 15.7549) centre (0, 0) ccw projected
  line L485 (44.2458, 16.1342) -> (43.2578, 15.7549) projected
  line L486 (45.5856, 17.0736) -> (44.2458, 16.1342) projected
  line L487 (45.3012, 17.8146) -> (45.5856, 17.0736) projected
  line L488 (43.6769, 17.6162) -> (45.3012, 17.8146) projected
  line L489 (42.6889, 17.2369) -> (43.6769, 17.6162) projected
  arc A111 (42.6889, 17.2369) -> (42.3739, 17.9972) centre (0, 0) ccw projected
  line L490 (43.3408, 18.4277) -> (42.3739, 17.9972) projected
  line L491 (44.6296, 19.4359) -> (43.3408, 18.4277) projected
  line L492 (44.3068, 20.1611) -> (44.6296, 19.4359) projected
  line L493 (42.6951, 19.8779) -> (44.3068, 20.1611) projected
  line L494 (41.7283, 19.4475) -> (42.6951, 19.8779) projected
  arc A112 (41.7283, 19.4475) -> (41.374, 20.1902) centre (0, 0) ccw projected
  line L495 (42.317, 20.6707) -> (41.374, 20.1902) projected
  line L496 (43.5512, 21.745) -> (42.317, 20.6707) projected
  line L497 (43.1909, 22.4523) -> (43.5512, 21.745) projected
  line L498 (41.5962, 22.0852) -> (43.1909, 22.4523) projected
  line L499 (40.6533, 21.6047) -> (41.5962, 22.0852) projected
  arc A113 (40.6533, 21.6047) -> (40.2606, 22.3279) centre (0, 0) ccw projected
  line L500 (41.1771, 22.8571) -> (40.2606, 22.3279) projected
  line L501 (42.3535, 23.9945) -> (41.1771, 22.8571) projected
  line L502 (41.9566, 24.6819) -> (42.3535, 23.9945) projected
  line L503 (40.3834, 24.2319) -> (41.9566, 24.6819) projected
  line L504 (39.4668, 23.7027) -> (40.3834, 24.2319) projected
  arc A114 (39.4668, 23.7027) -> (39.0369, 24.4044) centre (0, 0) ccw projected
  line L505 (39.9245, 24.9808) -> (39.0369, 24.4044) projected
  line L506 (41.0397, 26.1783) -> (39.9245, 24.9808) projected
  line L507 (40.6074, 26.844) -> (41.0397, 26.1783) projected
  line L508 (39.0598, 26.3122) -> (40.6074, 26.844) projected
  line L509 (38.1722, 25.7358) -> (39.0598, 26.3122) projected
  arc A115 (38.1722, 25.7358) -> (37.7061, 26.414) centre (0, 0) ccw projected
  line L510 (38.5623, 27.0361) -> (37.7061, 26.414) projected
  line L511 (39.6134, 28.2902) -> (38.5623, 27.0361) projected
  line L512 (39.1468, 28.9324) -> (39.6134, 28.2902) projected
  line L513 (37.6292, 28.3204) -> (39.1468, 28.9324) projected
  line L514 (36.773, 27.6983) -> (37.6292, 28.3204) projected
  arc A116 (36.773, 27.6983) -> (36.2721, 28.3512) centre (0, 0) ccw projected
  line L515 (37.0945, 29.0172) -> (36.2721, 28.3512) projected
  line L516 (38.0785, 30.3247) -> (37.0945, 29.0172) projected
  line L517 (37.579, 30.9415) -> (38.0785, 30.3247) projected
  line L518 (36.0955, 30.2509) -> (37.579, 30.9415) projected
  line L519 (35.273, 29.5849) -> (36.0955, 30.2509) projected
  arc A117 (35.273, 29.5849) -> (34.7386, 30.2107) centre (0, 0) ccw projected
  line L520 (35.5251, 30.9188) -> (34.7386, 30.2107) projected
  line L521 (36.4392, 32.276) -> (35.5251, 30.9188) projected
  line L522 (35.9081, 32.8659) -> (36.4392, 32.276) projected
  line L523 (34.4628, 32.0986) -> (35.9081, 32.8659) projected
  line L524 (33.6763, 31.3904) -> (34.4628, 32.0986) projected
  arc A118 (33.6763, 31.3904) -> (33.1099, 31.9873) centre (0, 0) ccw projected
  line L525 (33.8582, 32.7357) -> (33.1099, 31.9873) projected
  line L526 (34.7001, 34.1388) -> (33.8582, 32.7357) projected
  line L527 (34.1388, 34.7001) -> (34.7001, 34.1388) projected
  line L528 (32.7357, 33.8582) -> (34.1388, 34.7001) projected
  line L529 (31.9873, 33.1099) -> (32.7357, 33.8582) projected
  arc A119 (31.9873, 33.1099) -> (31.3904, 33.6763) centre (0, 0) ccw projected
  line L530 (32.0986, 34.4628) -> (31.3904, 33.6763) projected
  line L531 (32.8659, 35.9081) -> (32.0986, 34.4628) projected
  line L532 (32.276, 36.4392) -> (32.8659, 35.9081) projected
  line L533 (30.9188, 35.5251) -> (32.276, 36.4392) projected
  line L534 (30.2107, 34.7386) -> (30.9188, 35.5251) projected
  arc A120 (30.2107, 34.7386) -> (29.5849, 35.273) centre (0, 0) ccw projected
  line L535 (30.2509, 36.0955) -> (29.5849, 35.273) projected
  line L536 (30.9415, 37.579) -> (30.2509, 36.0955) projected
  line L537 (30.3247, 38.0785) -> (30.9415, 37.579) projected
  line L538 (29.0172, 37.0945) -> (30.3247, 38.0785) projected
  line L539 (28.3512, 36.2721) -> (29.0172, 37.0945) projected
  arc A121 (28.3512, 36.2721) -> (27.6983, 36.773) centre (0, 0) ccw projected
  line L540 (28.3204, 37.6292) -> (27.6983, 36.773) projected
  line L541 (28.9324, 39.1468) -> (28.3204, 37.6292) projected
  line L542 (28.2902, 39.6134) -> (28.9324, 39.1468) projected
  line L543 (27.0361, 38.5623) -> (28.2902, 39.6134) projected
  line L544 (26.414, 37.7061) -> (27.0361, 38.5623) projected
  arc A122 (26.414, 37.7061) -> (25.7358, 38.1722) centre (0, 0) ccw projected
  line L545 (26.3122, 39.0598) -> (25.7358, 38.1722) projected
  line L546 (26.844, 40.6074) -> (26.3122, 39.0598) projected
  line L547 (26.1783, 41.0397) -> (26.844, 40.6074) projected
  line L548 (24.9808, 39.9245) -> (26.1783, 41.0397) projected
  line L549 (24.4044, 39.0369) -> (24.9808, 39.9245) projected
  arc A123 (24.4044, 39.0369) -> (23.7027, 39.4668) centre (0, 0) ccw projected
  line L550 (24.2319, 40.3834) -> (23.7027, 39.4668) projected
  line L551 (24.6819, 41.9566) -> (24.2319, 40.3834) projected
  line L552 (23.9945, 42.3535) -> (24.6819, 41.9566) projected
  line L553 (22.8571, 41.1771) -> (23.9945, 42.3535) projected
  line L554 (22.3279, 40.2606) -> (22.8571, 41.1771) projected
  arc A124 (22.3279, 40.2606) -> (21.6047, 40.6533) centre (0, 0) ccw projected
  line L555 (22.0852, 41.5962) -> (21.6047, 40.6533) projected
  line L556 (22.4523, 43.1909) -> (22.0852, 41.5962) projected
  line L557 (21.745, 43.5512) -> (22.4523, 43.1909) projected
  line L558 (20.6707, 42.317) -> (21.745, 43.5512) projected
  line L559 (20.1902, 41.374) -> (20.6707, 42.317) projected
  arc A125 (20.1902, 41.374) -> (19.4475, 41.7283) centre (0, 0) ccw projected
  line L560 (19.8779, 42.6951) -> (19.4475, 41.7283) projected
  line L561 (20.1611, 44.3068) -> (19.8779, 42.6951) projected
  line L562 (19.4359, 44.6296) -> (20.1611, 44.3068) projected
  line L563 (18.4277, 43.3408) -> (19.4359, 44.6296) projected
  line L564 (17.9972, 42.3739) -> (18.4277, 43.3408) projected
  arc A126 (17.9972, 42.3739) -> (17.2369, 42.6889) centre (0, 0) ccw projected
  line L565 (17.6162, 43.6769) -> (17.2369, 42.6889) projected
  line L566 (17.8146, 45.3012) -> (17.6162, 43.6769) projected
  line L567 (17.0736, 45.5856) -> (17.8146, 45.3012) projected
  line L568 (16.1342, 44.2458) -> (17.0736, 45.5856) projected
  line L569 (15.7549, 43.2578) -> (16.1342, 44.2458) projected
  arc A127 (15.7549, 43.2578) -> (14.9792, 43.5325) centre (0, 0) ccw projected
  line L570 (15.3062, 44.539) -> (14.9792, 43.5325) projected
  line L571 (15.4193, 46.1715) -> (15.3062, 44.539) projected
  line L572 (14.6644, 46.4167) -> (15.4193, 46.1715) projected
  line L573 (13.7964, 45.0296) -> (14.6644, 46.4167) projected
  line L574 (13.4694, 44.023) -> (13.7964, 45.0296) projected
  arc A128 (13.4694, 44.023) -> (12.6803, 44.2568) centre (0, 0) ccw projected
  line L575 (12.9542, 45.279) -> (12.6803, 44.2568) projected
  line L576 (12.9818, 46.9152) -> (12.9542, 45.279) projected
  line L577 (12.2151, 47.1206) -> (12.9818, 46.9152) projected
  line L578 (11.4208, 45.6899) -> (12.2151, 47.1206) projected
  line L579 (11.1469, 44.6676) -> (11.4208, 45.6899) projected
  arc A129 (11.1469, 44.6676) -> (10.3467, 44.8597) centre (0, 0) ccw projected
  line L580 (10.5668, 45.895) -> (10.3467, 44.8597) projected
  line L581 (10.5086, 47.5303) -> (10.5668, 45.895) projected
  line L582 (9.7322, 47.6953) -> (10.5086, 47.5303) projected
  line L583 (9.0139, 46.225) -> (9.7322, 47.6953) projected
  line L584 (8.7939, 45.1898) -> (9.0139, 46.225) projected
  arc A130 (8.7939, 45.1898) -> (7.9848, 45.3398) centre (0, 0) ccw projected
  line L585 (8.1503, 46.3851) -> (7.9848, 45.3398) projected
  line L586 (8.0067, 48.0151) -> (8.1503, 46.3851) projected
  line L587 (7.2227, 48.1393) -> (8.0067, 48.0151) projected
  line L588 (6.5824, 46.6334) -> (7.2227, 48.1393) projected
  line L589 (6.4168, 45.5881) -> (6.5824, 46.6334) projected
  arc A131 (6.4168, 45.5881) -> (5.6009, 45.6955) centre (0, 0) ccw projected
  line L590 (5.7115, 46.7481) -> (5.6009, 45.6955) projected
  line L591 (5.4828, 48.3684) -> (5.7115, 46.7481) projected
  line L592 (4.6934, 48.4513) -> (5.4828, 48.3684) projected
  line L593 (4.1327, 46.914) -> (4.6934, 48.4513) projected
  line L594 (4.0221, 45.8615) -> (4.1327, 46.914) projected
  arc A132 (4.0221, 45.8615) -> (3.2017, 45.926) centre (0, 0) ccw projected
  line L595 (3.2571, 46.9829) -> (3.2017, 45.926) projected
  line L596 (2.9439, 48.589) -> (3.2571, 46.9829) projected
  line L597 (2.1512, 48.6306) -> (2.9439, 48.589) projected
  line L598 (1.6718, 47.066) -> (2.1512, 48.6306) projected
  line L599 (1.6164, 46.0091) -> (1.6718, 47.066) projected
  circle A133 centre (0, 0) radius 48.26
  dimension "d27" = 96.52
  constraints: 1 centre point, 1 coincident
  measures "d27" diameter of A133
body "Solid1"
